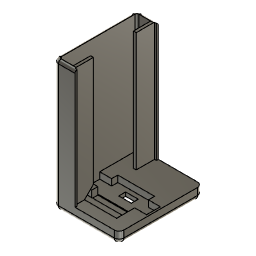
Person_Tracker (Autodesk Fusion 360 design; units mm, degrees)
Autodesk Fusion 360 part; units mm, degrees
sketch "Skizze1" plane through (0, 0, 0) normal (0, 0, 1) x (1, 0, 0)
  line L0 (0, 0) -> (15.5, 0)
  line L1 (15.5, 0) -> (15.5, -11)
  line L2 (15.5, -11) -> (0, -11)
  line L3 (0, -11) -> (0, 0)
  line L4 (15.5, -2.6) -> (20.5, -2.6)
  line L5 (20.5, -2.6) -> (20.5, -8.4)
  line L6 (20.5, -8.4) -> (15.5, -8.4)
  line L7 (15.5, -8.4) -> (15.5, -2.6)
  line L8 (0, -2.6) -> (-5, -2.6)
  line L9 (-5, -2.6) -> (-5, -8.4)
  line L10 (-5, -8.4) -> (0, -8.4)
  line L11 (0, -8.4) -> (0, -2.6)
  line L12 (5.1, -1.8) -> (10.4, -1.8)
  line L13 (10.4, -1.8) -> (10.4, -4.7)
  line L14 (10.4, -4.7) -> (5.1, -4.7)
  line L15 (5.1, -4.7) -> (5.1, -1.8)
  line L16 (7.75, 0) -> (7.75, -11) construction
  line L17 (0, -8.4) -> (15.5, -8.4)
  line L18 (-6.2, 14.25) -> (21.3, 14.25)
  line L19 (21.3, 14.25) -> (21.3, -20.75)
  line L20 (21.3, -20.75) -> (-6.2, -20.75)
  line L21 (-6.2, -20.75) -> (-6.2, 14.25)
  line L22 (10.4, -3.25) -> (5.1, -3.25) construction
  line L23 (-5, 13.05) -> (0.8, 13.05)
  line L24 (0.8, 13.05) -> (0.8, -19.55)
  line L25 (0.8, -19.55) -> (-5, -19.55)
  line L26 (-5, -19.55) -> (-5, 13.05)
  line L27 (0.8, 5.75) -> (2, 5.75)
  line L28 (2, 5.75) -> (2, 14.25)
  line L29 (0.8, -12.25) -> (2, -12.25)
  line L30 (2, -12.25) -> (2, -20.75)
  line L31 (2, 13.45) -> (2.8, 13.45)
  line L32 (2.8, 13.45) -> (2.8, 14.25)
  line L33 (2, -19.95) -> (2.8, -19.95)
  line L34 (2.8, -19.95) -> (2.8, -20.75)
  line L35 (15.5, -11) -> (15.5, -16)
  line L36 (15.5, -16) -> (-2.5, -16)
  line L37 (-2.5, -16) -> (-2.5, -11)
  line L38 (-2.5, -11) -> (0, -11)
  dimension "d1" = 15.5
  dimension "d2" = 11
  dimension "d3" = 5
  dimension "d4" = 5.8
  dimension "d5" = 5
  dimension "d6" = 5.8
  dimension "d7" = 5.3
  dimension "d8" = 2.9
  dimension "d9" = 1.8
  dimension "d10" = 2.65
  dimension "d42" = 35
  dimension "d43" = 17.5
  dimension "d44" = 0.8
  dimension "d45" = 1.2
  dimension "d46" = 1.2
  dimension "d47" = 1.2
  dimension "d48" = 5.8
  dimension "d49" = 1.2
  dimension "d51" = 8.5
  dimension "d52" = 8.5
  dimension "d53" = 1.2
  dimension "d55" = 0.8
  dimension "d56" = 0.8
  dimension "d57" = 0.8
  dimension "d58" = 0.8
  dimension "d59" = 18.4
  dimension "d66" = 18
  dimension "d67" = 5
  constraint horizontal L0
  constraint vertical L1
  constraint horizontal L2
  constraint vertical L3
  constraint coincident L0.start L3.end
  constraint horizontal L4
  constraint vertical L5
  constraint horizontal L6
  constraint vertical L7
  constraint coincident L1 L4.start
  constraint horizontal L8
  constraint vertical L9
  constraint horizontal L10
  constraint vertical L11
  constraint coincident L3 L8.start
  constraint midpoint L3 L11
  constraint midpoint L1 L7
  constraint horizontal L12
  constraint vertical L13
  constraint horizontal L14
  constraint vertical L15
  constraint midpoint L0 L16.start
  constraint midpoint L2 L16.end
  constraint coincident L3 L10.end
  constraint coincident L1 L6.end
  constraint perpendicular L1 L17
  constraint collinear L6 L17
  constraint horizontal L18
  constraint vertical L19
  constraint horizontal L20
  constraint vertical L21
  constraint midpoint L13 L22.start
  constraint midpoint L15 L22.end
  constraint horizontal L23
  constraint vertical L24
  constraint horizontal L25
  constraint vertical L26
  constraint coincident L24 L27.start
  constraint perpendicular L24 L27
  constraint coincident L18 L28.end
  constraint perpendicular L18 L28
  constraint coincident L24 L29.start
  constraint perpendicular L24 L29
  constraint coincident L20 L30.end
  constraint perpendicular L20 L30
  constraint collinear L28 L30
  constraint coincident L28 L31.start
  constraint perpendicular L28 L31
  constraint coincident L18 L32.end
  constraint perpendicular L18 L32
  constraint coincident L30 L33.start
  constraint perpendicular L30 L33
  constraint coincident L20 L34.end
  constraint perpendicular L20 L34
  constraint perpendicular L2 L35
  constraint perpendicular L24 L36
  constraint perpendicular L36 L37
  constraint collinear L2 L38
  measures "d1" distance of L0.start L0.end
  measures "d2" distance of L0.start L2.end
  measures "d3" distance of L4.start L4.end
  measures "d4" distance of L4.start L6.end
  measures "d5" distance of L8.start L8.end
  measures "d6" distance of L8.start L10.end
  measures "d7" distance of L12.start L12.end
  measures "d8" distance of L12.start L14.end
  measures "d9" distance of L0 L12
  measures "d10" distance of L13 L16
  measures "d42" distance of L18.start L20.end
  measures "d43" distance of L18 L22
  measures "d44" distance of L5 L19
  measures "d45" distance of L20 L25
  measures "d46" distance of L18 L23
  measures "d47" distance of L21 L26
  measures "d48" distance of L24 L26
  measures "d49" distance of L9 L21
  measures "d51" distance of L27.end L28.end
  measures "d52" distance of L29.end L30.end
  measures "d53" distance of L24 L30
  measures "d55" distance of L33.start L33.end
  measures "d56" distance of L33.end L34.end
  measures "d57" distance of L31.end L32.end
  measures "d58" distance of L28 L32
  measures "d66" distance of L35 L37
  measures "d67" distance of L2 L36
extrude "Extrusion1" add sketch "Skizze1" along normal blind 1.8 contours L2 L3 L17 L24 | L1 L2 L17 L24
extrude "Extrusion2" add sketch "Skizze1" along normal blind 2.2 contours L0 L3 L11 L17 L24 | L0 L1 L7 L17 L24 | L3 L8 L9 L10 L11 L26 | L1 L4 L5 L6 L7 | L2 L24 L36 L37 L38 | L2 L24 L29 L30 L35 L36 | L24 L29 L30 L36
extrude "Extrusion3" add sketch "Skizze1" along normal blind 4.9 contours L0 L3 L8 L23 L24 L26 | L0 L1 L4 L5 L6 L18 L19 L20 L24 L27 L28 L30 L31 L32 L33 L34 L35 L36 | L9 L18 L20 L21 L23 L24 L25 L26 L27 L28 L30 L36 | L3 L10 L24 L25 L26 L36 L37 L38 | L18 L28 L31 L32 | L20 L30 L33 L34
extrude "Extrusion4" add sketch "Skizze1" along normal blind 50 from surface at 4.9 contours L9 L18 L20 L21 L23 L24 L25 L26 L27 L28 L30 L36 | L18 L28 L31 L32 | L24 L29 L30 L36 | L20 L30 L33 L34
chamfer "Fase1" distance 0.6 angle 45 4 edges at (7.75, -4.7, 0) (5.1, -3.25, 0) (7.75, -1.8, 0) (10.4, -3.25, 0)
fillet "Abrundung1" radius 0.8 2 edges at (-5, 13.05, 29.9) (-5, -19.55, 29.9)
fillet "Abrundung2" radius 2 8 edges at (-6.2, 14.25, 27.45) (-6.2, -20.75, 27.45) (-6.2, -3.25, 0) (7.55, 14.25, 0) (21.3, 14.25, 2.45) (21.3, -20.75, 2.45) (21.3, -3.25, 0) (7.55, -20.75, 0)
fillet "Abrundung3" radius 1.2 5 edges at (-0.7, 14.25, 54.9) (-5.6142, 13.6642, 54.9) (-6.2, -3.25, 54.9) (-5.6142, -20.1642, 54.9) (-0.7, -20.75, 54.9)
chamfer "Fase2" distance 3.75 angle 45 1 edges at (1.4, -12.25, 4.9)
equation "d10 = ( 5.3 / 2 ) * 1 mm"
equation "d29 = 0.6 mm + 1.6 mm + 2.7 mm"
equation "d43 = ( 35 / 2 ) * 1 mm"
equation "d51 = ( ( 35 - 18 ) / 2 ) * 1 mm"
equation "d52 = ( ( 35 - 18 ) / 2 ) * 1 mm"
equation "d61 = 2 mm - 1.2 mm"
equation "d68 = 0.6 mm + 1.6 mm + 2.7 mm"
named bodies: "Person_Tracker"
